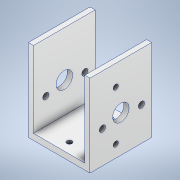
# Autodesk Inventor part: hand1
Saved by Autodesk Inventor 2022 (Build 260153000, 153)
## iProperties
Created: 2022-04-20
Part Number: hand1
Material: アルミニウム 6061
Document SubType Name: Modeling
Designer: Yazawa
Density: 2.7 g/cm^3
Appearance: アルミニウム - フラット
Author: Yazawa
Autodesk Inventor part; units mm, degrees
ref_plane "YZ Plane" through (0, 0, 0) normal (1, 0, 0) x (0, 1, 0)
ref_plane "XZ Plane" through (0, 0, 0) normal (0, 1, 0) x (-1, 0, 0)
sketch "スケッチ1" plane through (0, 0, 0) normal (0, 1, 0) x (-1, 0, 0)
  line L0 (15, -15) -> (-15, -15)
  line L1 (-15, -15) -> (-15, 15)
  line L2 (-15, 15) -> (15, 15)
  line L3 (15, 15) -> (15, -15)
  line L4 (-15, 15) -> (15, -15) construction
  line L5 (-15, -15) -> (15, 15) construction
  point P0 (0, 0)
  point P1 (0, 0)
  dimension "d0" = 30
  dimension "d1" = 30
  constraints: 12 end point, 2 midpoint, 2 parallel, 1 coincident, 1 horizontal, 1 perpendicular
  measures "d0" distance of L1.end L2.end
  measures "d1" distance of L0.end L1.end
extrude "押し出し1" add sketch "スケッチ1" along normal blind 3
sketch "スケッチ2" plane through (0, 3, 0) normal (0, 1, 0) x (1, 0, 0)
  line L0 (-15, -15) -> (15, -15) projected
  line L1 (15, -15) -> (15, 15) projected
  line L2 (15, 15) -> (-15, 15) projected
  line L3 (-15, 15) -> (-15, -15) projected
  line L4 (-15, -15) -> (15, -15) projected
  line L5 (-15, -15) -> (-12.5, -15)
  line L6 (-12.5, -15) -> (-12.5, 15)
  line L7 (-12.5, 15) -> (-15, 15)
  line L8 (-15, 15) -> (-15, -15)
  line L9 (15, -15) -> (15, 15) projected
  line L10 (15, -15) -> (12.5, -15)
  line L11 (12.5, -15) -> (12.5, 15)
  line L12 (12.5, 15) -> (15, 15)
  line L13 (15, 15) -> (15, -15)
  line L14 (15, 15) -> (-15, 15) projected
  point P0 (0, 0)
  point P1 (-12.5, 15)
  dimension "d4" = 2.5
  dimension "d5" = 2.5
  constraints: 16 end point, 4 parallel, 2 collinear, 2 horizontal, 2 perpendicular
  measures "d4" distance of L7.end L6.end
  measures "d5" distance of L11.end L12.end
extrude "押し出し2" add sketch "スケッチ2" along normal blind 40 from surface at -3 contours L3 L2 L6 L0 | L11 L2 L1 L0
sketch "スケッチ3" plane through (15, 0, 15) normal (1, 0, 0) x (0, 0, -1)
  line L0 (0, 3) -> (30, 3) projected
  line L1 (15, 18) -> (30, 18) construction
  line L2 (30, 40) -> (30, 3) construction
  line L3 (15, 18) -> (-10.0782, 18) construction
  point P0 (15, 0)
  dimension "d8" = 15
  dimension "d50" = 15
  constraints: 4 end point, 2 point on line, 1 horizontal
  measures "d8" distance from line of L0 L1.start
  measures "d50" distance of L1.start L1.end
hole "穴1" at (15, 18, 0) direction (-1, 0, 0) diameter 8 end through all
sketch "スケッチ6" plane through (0, 3, 0) normal (0, 1, 0) x (1, 0, 0)
  line L0 (12.5, 15) -> (-12.5, 15) projected
  point P0 (0, 0)
  point P1 (0, 10)
  point P2 (0, -10)
  point P3 (0, 15)
  dimension "d41" = 5
  dimension "d42" = 20
  constraints: 2 vertical alignment, 1 midpoint
  measures "d41" distance from line of L0 point (0, 10)
  measures "d42" distance of point (0, -10) point (0, 10)
hole "穴3" at (0, 3, -10) at (0, 3, 10) direction (0, -1, 0) diameter 2.459 depth 3 thread size "M3x0.5" class "6H" standard "ISO Metric profile"
sketch "スケッチ8" plane through (15, 0, 15) normal (1, 0, 0) x (0, 0, -1)
  circle A0 centre (15, 18) radius 4 projected
  line L0 (12.5, 30) -> (12.5, 6) construction
  point P0 (15, 0)
  dimension "d56" = 24
  dimension "d57" = 12
  dimension "d58" = 2.5
  constraints: 2 coincident, 2 end point, 1 vertical
  measures "d56" distance of L0.start L0.end
  measures "d57" vertical distance of A0.centre L0.start
  measures "d58" distance from line of L0 A0.centre
hole "穴4" at (15, 30, 2.5) at (15, 6, 2.5) direction (-1, 0, 0) diameter 2.459 depth 2.5 thread size "M3x0.5" class "6H" standard "ISO Metric profile"
sketch "スケッチ9" plane through (15, 0, 15) normal (1, 0, 0) x (0, 0, -1)
  circle A0 centre (15, 18) radius 4 projected
  line L0 (0, 18) -> (15, 18)
  line L1 (0, 0) -> (0, 40) projected
  line L2 (30, 0) -> (30, 40) projected
  line L3 (15, 18) -> (-5.0402, 29.5702)
  line L4 (15, 18) -> (33.9658, 28.9499)
  circle A1 centre (6, 15.6906) radius 1.5
  circle A2 centre (25, 16.2679) radius 1.5
  line L5 (12.5, 13.6699) -> (-5.7345, 24.1976)
  line L6 (17.5, 13.6699) -> (25.6852, 18.3956)
  point P0 (15, 0)
  dimension "d70" = 3
  dimension "d71" = 3
  dimension "d72" = 6
  dimension "d73" = 5
  dimension "d83" = 5
  dimension "d84" = 5
  dimension "d85" = 30
  dimension "d86" = 30
  constraints: 11 end point, 2 centre point, 2 coincident, 2 parallel, 2 tangent, 1 horizontal, 1 point on line
  measures "d70" diameter of A2
  measures "d71" diameter of A1
  measures "d72" distance from line of L1 A1.centre
  measures "d73" distance from line of L2 A2.centre
  measures "d83" distance between parallel lines of L3 L5
  measures "d84" distance between parallel lines of L4 L6
  measures "d85" angle of L3 L0
  measures "d86" angle of L4 L0
hole "穴5" at (15, 15.6906, 9) at (15, 16.2679, -10) direction (-1, 0, 0) diameter 3 depth 30
ref_plane "作業平面1" through (0, 3, 15) normal (1, 0, 0) x (0, 0, -1)
